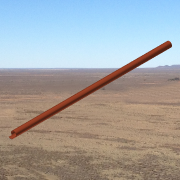
# Autodesk Inventor part: 2f1arm
Saved by Autodesk Inventor 2013 SP2 (Build 170200200, 200)
## iProperties
Company: HERA Project
Created: 2013-05-22
Part Number: 2f1arm
Material: Copper
Document SubType Name: Modeling
Designer: Dave
Density: 8.94 g/cm^3
Description: Feed arm pipe
Mass: 433.292 g
Surface Area: 850.1 cm^2
Volume: 48.4666 cm^3
Translation Standard: STEP AP214IS
FileName: C:/Users/Dave/Desktop/PAPER/paperElement.step
PostProcessor: Build: 138, Release: 2013 RTM - Date: Thu 03/01/2012
Sent Units: centimeter
Uncertainty: 0.0
Author: David DeBoer
Title: Feed arm
Autodesk Inventor part; units mm, degrees
ref_plane "YZ Plane" through (0, 0, 0) normal (1, 0, 0) x (0, 1, 0)
ref_plane "XZ Plane" through (0, 0, 0) normal (0, 1, 0) x (-1, 0, 0)
ref_plane "XY Plane" through (0, 0, 0) normal (0, 0, 1) x (1, 0, 0)
sketch "Sketch1" plane through (0, 0, 0) normal (0, 0, 1) x (1, 0, 0)
  circle A0 centre (0, 0) radius 11.1125
  circle A1 centre (-0.2084, 0) radius 9.9695
  dimension "d0" = 22.225
  dimension "d2" = 19.939
  constraints: 2 centre point, 1 coincident
  measures "d0" diameter of A0
  measures "d2" diameter of A1
extrude "Extrusion1" add sketch "Sketch1" along normal blind 649.986
sketch "Sketch2" plane through (0, 0, 649.986) normal (0, 0, 1) x (1, 0, 0)
  line L0 (-12.7, -7.6835) -> (12.3613, -7.6835)
  line L1 (12.3613, -7.6835) -> (12.3613, 11.1125)
  line L2 (12.3613, 11.1125) -> (-12.7, 11.1125)
  line L3 (-12.7, 11.1125) -> (-12.7, -7.6835)
  dimension "d5" = 18.796
  constraints: 8 end point, 2 parallel, 1 horizontal, 1 perpendicular
  measures "d5" distance of L2.end L0.start
extrude "Extrusion2" cut sketch "Sketch2" against normal blind 12.7
sketch "Sketch3" plane through (0, 0, 649.986) normal (0, 0, 1) x (1, 0, 0)
  line L0 (8.0282, -7.6835) -> (6.1441, -7.6835) projected
  arc A0 (-6.561, -7.6835) -> (6.1441, -7.6835) centre (-0.2084, 0) ccw projected
  line L1 (-6.561, -7.6835) -> (-8.0282, -7.6835) projected
  arc A1 (-8.0282, -7.6835) -> (8.0282, -7.6835) centre (0, 0) ccw projected
  point P0 (0, -11.1125)
  constraints: 1 point on circle
ref_plane "Work Plane1" through (0, -11.1125, 649.986) normal (0, -1, 0) x (1, 0, 0)
sketch "Sketch4" plane through (0, -11.1125, 649.986) normal (0, -1, 0) x (1, 0, 0)
  circle A0 centre (0, -2.032) radius 1.4732
  line L0 (8.0282, 0) -> (-8.0282, 0) projected
  point P0 (0, -649.986)
  dimension "d9" = 2.9464
  dimension "d11" = 2.032
  constraints: 1 centre point
  measures "d9" diameter of A0
  measures "d11" distance from line of A0.centre L0
extrude "Extrusion3" cut sketch "Sketch4" against normal blind 12.7
body "Solid2"
